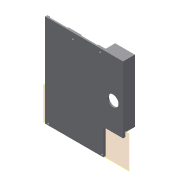
# Autodesk Inventor part: 10_MiniSPIM_Lid
Saved by Autodesk Inventor 2019 (Build 230136000, 136)
## iProperties
Created: 2019-10-13
Part Number: 10_MiniSPIM_Lid
Material: Generic
Document SubType Name: Modeling
Designer: diederichbenedict
Density: 1 g/cm^3
Appearance: Default
Author: diederichbenedict
Autodesk Inventor part; units mm, degrees
ref_plane "YZ Plane" through (0, 0, 0) normal (1, 0, 0) x (0, 1, 0)
ref_plane "XZ Plane" through (0, 0, 0) normal (0, 1, 0) x (-1, 0, 0)
ref_plane "Work Plane1" through (0, 0, 0) normal (0, 0, 1) x (1, 0, 0)
sketch "Sketch1" plane through (0, 0, 0) normal (0, 0, 1) x (1, 0, 0)
  circle A0 centre (-49.8552, -60.9647) radius 1.65 construction
  circle A1 centre (24.2311, -60.9647) radius 1.65 construction
  arc A2 (22.7622, -32.9022) -> (21.5, -36.5843) centre (37.7579, -40.1) ccw construction
  line L0 (22.7622, -32.9022) -> (25.7, -32.9022) construction
  line L1 (25.7, -32.9022) -> (25.7, -35.65) construction
  arc A3 (25.7, -44.55) -> (25.7, -35.65) centre (2.4892, -40.1) ccw construction
  line L2 (25.7, -44.55) -> (25.7, -47.2978) construction
  line L3 (25.7, -47.2978) -> (22.7622, -47.2978) construction
  arc A4 (21.5, -43.6157) -> (22.7622, -47.2978) centre (37.7579, -40.1) ccw construction
  line L4 (21.5, -58.1715) -> (21.5, -43.6157) construction
  line L5 (-53.5, -58.1715) -> (21.5, -58.1715) construction
  line L6 (-53.5, -63.7578) -> (-53.5, -58.1715) construction
  line L7 (26.5, -63.7578) -> (-53.5, -63.7578) construction
  line L8 (26.5, -27.7578) -> (26.5, -63.7578) construction
  line L9 (53.5, -27.7578) -> (26.5, -27.7578) construction
  line L10 (53.5, -22.7578) -> (53.5, -27.7578) construction
  line L11 (21.5, -22.7578) -> (53.5, -22.7578) construction
  line L12 (21.5, -36.5843) -> (21.5, -22.7578) construction
  line L13 (21.5, -39.9422) -> (21.5, 19.8578) construction
  line L14 (26.5, 63.7578) -> (26.5, 13.7578) construction
  line L15 (16.5, 20.8578) -> (16.5, 63.7578) construction
  line L16 (-6.7098, 63.7578) -> (-6.7098, 48.6857) construction
  line L17 (-24.537, 20.8578) -> (-24.537, 63.7578) construction
  line L18 (-49.8552, 63.7578) -> (-49.8552, 20.8578) construction
  line L19 (-53.5, 63.7578) -> (-53.5, -63.7578) construction
  line L20 (-53.5, -63.7578) -> (26.5, -63.7578)
  line L21 (26.5, -63.7578) -> (26.5, -58.1715)
  line L22 (26.5, -58.1715) -> (-53.5, -58.1715)
  line L23 (-53.5, -58.1715) -> (-53.5, -63.7578)
  line L24 (21.5, -58.1715) -> (26.5, -58.1715)
  line L25 (26.5, -58.1715) -> (26.5, 20.8578)
  line L26 (26.5, 20.8578) -> (21.5, 20.8578)
  line L27 (21.5, 20.8578) -> (21.5, -58.1715)
  line L28 (16.5, 20.8578) -> (26.5, 20.8578)
  line L29 (26.5, 20.8578) -> (26.5, 63.7578)
  line L30 (26.5, 63.7578) -> (16.5, 63.7578)
  line L31 (16.5, 63.7578) -> (16.5, 20.8578)
  line L32 (-49.8552, 63.7578) -> (-24.537, 63.7578)
  line L33 (-24.537, 63.7578) -> (-24.537, 20.8578)
  line L34 (-24.537, 20.8578) -> (-49.8552, 20.8578)
  line L35 (-49.8552, 20.8578) -> (-49.8552, 63.7578)
  line L36 (26.6067, -27.7578) -> (53.5, -27.7578)
  line L37 (53.5, -27.7578) -> (53.5, -22.7578)
  line L38 (53.5, -22.7578) -> (26.6067, -22.7578)
  line L39 (26.6067, -22.7578) -> (26.6067, -27.7578)
  line L40 (-6.7098, 63.7578) -> (-24.537, 63.7578)
  line L41 (-24.537, 63.7578) -> (-24.537, 48.6857)
  line L42 (-24.537, 48.6857) -> (-6.7098, 48.6857)
  line L43 (-6.7098, 48.6857) -> (-6.7098, 63.7578)
  circle A5 centre (21.5, 59.4877) radius 1.65 projected
  circle A6 centre (24.2311, -60.9647) radius 1.65 projected
  circle A7 centre (-49.8552, -60.9647) radius 1.65 projected
  circle A8 centre (-16, 56.2217) radius 1.65 projected
  line L44 (-53.5, 63.7578) -> (-49.8552, 63.7578)
  line L45 (-49.8552, 63.7578) -> (-49.8552, 20.8578)
  line L46 (-49.8552, 20.8578) -> (-53.5, 20.8578)
  line L47 (-53.5, 20.8578) -> (-53.5, 63.7578)
  circle A9 centre (21.5, 27.3048) radius 1.65 projected
  point P0 (0, 0)
  constraints: 56 end point, 14 parallel, 7 horizontal, 7 perpendicular, 4 point on line
extrude "Extrusion1" add sketch "Sketch1" along normal blind 1.1 contours L23 L22 L21 L20 | L22 L27 L26 L25 | L26 L28 L31 L30 L29 | L35 L46 L47 L44 | L40 L43 L42 L33 | L39 L38 L37 L36
sketch "Sketch2" plane through (0, 0, 1.1) normal (0, 0, 1) x (1, 0, 0)
  circle A0 centre (-49.8552, -60.9647) radius 1.65 projected
  circle A1 centre (24.2311, -60.9647) radius 1.65 projected
  circle A2 centre (21.5, 59.4877) radius 1.65 projected
  line L0 (26.5, -63.7578) -> (26.5, 63.7578) projected
  line L1 (26.5, 63.7578) -> (16.5, 63.7578) projected
  line L2 (16.5, 63.7578) -> (16.5, 20.8578) projected
  line L3 (16.5, 20.8578) -> (21.5, 20.8578) projected
  line L4 (21.5, 20.8578) -> (21.5, -58.1715) projected
  line L5 (21.5, -58.1715) -> (-53.5, -58.1715) projected
  line L6 (-53.5, -58.1715) -> (-53.5, -63.7578) projected
  line L7 (-53.5, -63.7578) -> (26.5, -63.7578) projected
  line L8 (-49.8552, 63.7578) -> (-49.8552, 20.8578) projected
  line L9 (-6.7098, 63.7578) -> (-49.8552, 63.7578) projected
  line L10 (21.5, 20.8578) -> (16.5, 20.8578) projected
  line L11 (-49.8552, 63.7578) -> (16.5, 63.7578)
  line L12 (16.5, 63.7578) -> (16.5, 20.8578)
  line L13 (16.5, 20.8578) -> (-49.8552, 20.8578)
  line L14 (-49.8552, 20.8578) -> (-49.8552, 63.7578)
  line L15 (21.5, -58.1715) -> (-53.5, -58.1715) projected
  line L16 (-49.8552, 20.8578) -> (21.5, 20.8578)
  line L17 (21.5, 20.8578) -> (21.5, -58.1715)
  line L18 (21.5, -58.1715) -> (-49.8552, -58.1715)
  line L19 (-49.8552, -58.1715) -> (-49.8552, 20.8578)
  line L20 (-53.5, -58.1715) -> (-49.8552, -58.1715)
  line L21 (-49.8552, -58.1715) -> (-49.8552, 63.7578)
  line L22 (-49.8552, 63.7578) -> (-53.5, 63.7578)
  line L23 (-53.5, 63.7578) -> (-53.5, -58.1715)
  line L24 (53.5, -27.7578) -> (53.5, -22.7578) projected
  line L25 (26.5, 63.7578) -> (53.5, 63.7578)
  line L26 (53.5, 63.7578) -> (53.5, -27.7578)
  line L27 (53.5, -27.7578) -> (26.5, -27.7578)
  line L28 (26.5, -27.7578) -> (26.5, 63.7578)
  circle A3 centre (21.5, 59.4877) radius 1.65 projected
  circle A4 centre (-16, 56.2217) radius 1.65 projected
  line L29 (16.5, 63.7578) -> (16.5, 20.8578) projected
  line L30 (16.5, 63.7578) -> (26.5, 63.7578)
  circle A5 centre (24.2311, -60.9647) radius 1.65 projected
  line L31 (16.5, 20.8578) -> (-49.8552, 20.8578)
  line L32 (-49.8552, 20.8578) -> (-49.8552, 63.7578)
  line L33 (-49.8552, 63.7578) -> (16.5, 63.7578)
  line L34 (16.5, 63.7578) -> (16.5, 20.8578)
  ellipse E0 centre (39.7, 10.0578) end of major axis (44.7, 10.0578) minor radius 3.5355 projected
  circle A6 centre (39.7, 10.0578) radius 7.5
  circle A7 centre (21.5, 27.3048) radius 1.65 projected
  point P0 (0, 0)
  dimension "d4" = 15
  constraints: 42 end point, 10 parallel, 6 perpendicular, 5 horizontal, 1 centre point, 1 coincident, 1 other
  measures "d4" diameter of A6
extrude "Extrusion2" add sketch "Sketch2" along normal blind 2 contours L7 L6 L5 L4 L3 L2 L1 L0 | L0 L25 L26 L24 L27 | L23 L22 L8 L19 L5 | L2 L13 L8 L9 L11 | L19 L13 L3 L4 L5
ref_plane "Work Plane2" through (26.5, 18.8696, -13.1) normal (0, 0, 1) x (1, 0, 0)
sketch "Sketch3" plane through (0, 0, 1.1) normal (0, 0, -1) x (-1, 0, 0)
  circle A0 centre (16, 56.2217) radius 1.65 projected
  circle A1 centre (-39.7, 10.0578) radius 7.5 projected
  circle A2 centre (-21.5, 59.4877) radius 1.65 projected
  circle A3 centre (-24.2311, -60.9647) radius 1.65 projected
  circle A4 centre (49.8552, -60.9647) radius 1.65 projected
  line L0 (-53.5, 63.7578) -> (53.5, 63.7578) projected
  line L1 (53.5, 63.7578) -> (53.5, -63.7578) projected
  line L2 (53.5, -63.7578) -> (-26.5, -63.7578) projected
  line L3 (-26.5, -63.7578) -> (-26.5, -27.7578) projected
  line L4 (-26.5, -27.7578) -> (-53.5, -27.7578) projected
  line L5 (-53.5, -27.7578) -> (-53.5, 63.7578) projected
  line L6 (-26.5, 18.8696) -> (-45, 18.8696) projected
  line L7 (-45, 18.8696) -> (-45, 63.7578) projected
  line L8 (-45, 63.7578) -> (-26.5, 63.7578) projected
  line L9 (-26.5, 63.7578) -> (-26.5, 18.8696) projected
  line L10 (-70.915, -41.1304) -> (-130.915, -41.1304) projected
  line L11 (-130.915, -41.1304) -> (-130.915, 18.8696) projected
  line L12 (-130.915, 18.8696) -> (-45, 18.8696) projected
  line L13 (-45, 18.8696) -> (-45, 5.872) projected
  line L14 (-45, 5.872) -> (-26.5, 5.872) projected
  line L15 (-26.5, 5.872) -> (-26.5, 13.7578) projected
  line L16 (-26.5, 13.7578) -> (-21.5, 13.7578) projected
  line L17 (-21.5, 13.7578) -> (-21.5, 19.8578) projected
  line L18 (-21.5, 19.8578) -> (53.5, 19.8578) projected
  line L19 (53.5, 19.8578) -> (53.5, -58.1715) projected
  line L20 (53.5, -58.1715) -> (-21.5, -58.1715) projected
  line L21 (-21.5, -58.1715) -> (-21.5, -39.9578) projected
  line L22 (-21.5, -39.9578) -> (-21.5, -22.7578) projected
  line L23 (-21.5, -22.7578) -> (-28.8534, -22.7578) projected
  line L24 (-28.8534, -22.7578) -> (-28.8534, -2.7892) projected
  line L25 (-28.8534, -2.7892) -> (-50.0866, -2.7892) projected
  line L26 (-50.0866, -2.7892) -> (-50.0866, -22.7578) projected
  line L27 (-50.0866, -22.7578) -> (-53.5, -22.7578) projected
  line L28 (-53.5, -22.7578) -> (-53.5, -27.7578) projected
  line L29 (-53.5, -27.7578) -> (-70.915, -27.7578) projected
  line L30 (-70.915, -27.7578) -> (-70.915, -41.1304) projected
  circle A5 centre (-125.915, -11.1304) radius 2.95 projected
  circle A6 centre (-125.915, -36.1304) radius 2.95 projected
  circle A7 centre (-100.915, -36.1304) radius 2.95 projected
  circle A8 centre (-75.915, -36.1304) radius 2.95 projected
  circle A9 centre (-75.915, -11.1304) radius 2.95 projected
  circle A10 centre (-75.915, 13.8696) radius 2.95 projected
  circle A11 centre (-100.915, 13.8696) radius 2.95 projected
  circle A12 centre (-125.915, 13.8696) radius 2.95 projected
  line L31 (-53.5, 63.7578) -> (53.5, 63.7578) projected
  line L32 (-53.5, 63.7578) -> (-50.5, 63.7578)
  line L33 (-50.5, 63.7578) -> (-50.5, -22.2422)
  line L34 (-50.5, -22.2422) -> (-53.5, -22.2422)
  line L35 (-53.5, -22.2422) -> (-53.5, 63.7578)
  line L36 (-50.5, 63.7578) -> (-26.5, 63.7578)
  line L37 (-26.5, 63.7578) -> (-26.5, 60.7578)
  line L38 (-26.5, 60.7578) -> (-50.5, 60.7578)
  line L39 (-50.5, 60.7578) -> (-50.5, 63.7578)
  line L40 (-16.5, 63.7578) -> (-26.5, 63.7578) projected
  line L41 (-50.5, 60.7578) -> (-26.5, 60.7578)
  line L42 (-26.5, 60.7578) -> (-26.5, 63.7578)
  line L43 (-26.5, 63.7578) -> (-50.5, 63.7578)
  line L44 (-50.5, 63.7578) -> (-50.5, 60.7578)
  point P0 (0, 0)
  dimension "d5" = 3
  dimension "d6" = 86
  dimension "d7" = 3
  constraints: 24 end point, 6 parallel, 3 horizontal, 3 perpendicular, 1 point on line
  measures "d5" distance of L33.end L34.end
  measures "d6" distance of L32.end L33.end
  measures "d7" distance of L36.end L37.end
extrude "Extrusion3" add sketch "Sketch3" along normal up to surface (14.2 mm away) contours L38 L33 L0 L7 | L7 L0 L9 L38 | L33 L34 L5 L12 | L12 L5 L0 L33
body "Solid1"
